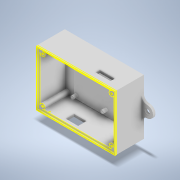
# Autodesk Inventor part: esp_housing_dsrm
Saved by Autodesk Inventor 2022.2 (Build 262287030, 287C)
## iProperties
Created: 2023-01-11
Part Number: esp_housing_dsrm
Material: Generic
Document SubType Name: Modeling
Designer: Ritchie
Density: 1 g/cm^3
Appearance: Default
Author: Ritchie
Autodesk Inventor part; units mm, degrees
ref_plane "YZ Plane" through (0, 0, 0) normal (1, 0, 0) x (0, 1, 0)
ref_plane "XZ Plane" through (0, 0, 0) normal (0, 1, 0) x (-1, 0, 0)
ref_plane "XY Plane" through (0, 0, 0) normal (0, 0, 1) x (1, 0, 0)
sketch "Sketch1" plane through (0, 0, 0) normal (0, 0, 1) x (1, 0, 0)
  line L0 (0, 0) -> (65.024, 0)
  line L1 (65.024, 0) -> (65.024, 56.742)
  line L2 (65.024, 56.742) -> (0, 56.742)
  line L3 (0, 56.742) -> (0, 0)
  point P0 (2.746, 53.796)
  point P1 (62.746, 53.796)
  point P2 (62.746, 3.796)
  point P3 (2.746, 3.796)
  point P4 (38.746, 53.796)
  point P5 (38.746, 6.796)
  dimension "d0" = 56.742
  dimension "d1" = 65.024
  dimension "d2" = 53.796
  dimension "d3" = 2.746
  dimension "d4" = 62.746
  dimension "d5" = 3.796
  dimension "d6" = 38.746
  dimension "d7" = 6.796
  dimension "d8" = 53.796
  dimension "d9" = 38.746
  constraints: 8 end point, 2 horizontal alignment, 2 parallel, 2 vertical alignment, 1 horizontal, 1 perpendicular
  measures "d0" distance of L2.end L0.start
  measures "d1" distance of L1.end L2.end
  measures "d2" distance from line of point (2.746, 53.796) L0
  measures "d3" distance from line of L3 point (2.746, 53.796)
  measures "d4" distance from line of L3 point (62.746, 53.796)
  measures "d5" distance from line of L0 point (2.746, 3.796)
  measures "d6" distance from line of point (38.746, 6.796) L3
  measures "d7" distance from line of L0 point (38.746, 6.796)
  measures "d8" distance from line of L0 point (38.746, 53.796)
  measures "d9" distance from line of L3 point (38.746, 53.796)
extrude "Extrusion1" add sketch "Sketch1" along normal blind 4
sketch "Sketch2" plane through (0, 0, 4) normal (0, 0, 1) x (1, 0, 0)
  circle A0 centre (2.746, 53.796) radius 2
  circle A1 centre (62.746, 53.796) radius 2
  circle A2 centre (38.746, 53.796) radius 2
  circle A3 centre (38.746, 6.796) radius 2
  circle A4 centre (2.746, 3.796) radius 2
  circle A5 centre (62.746, 3.796) radius 2
  point P0 (0, 0)
  dimension "d12" = 4
  dimension "d13" = 4
  dimension "d14" = 4
  dimension "d15" = 4
  dimension "d16" = 4
  dimension "d17" = 4
  constraints: 6 centre point, 6 coincident
  measures "d12" diameter of A0
  measures "d13" diameter of A1
  measures "d14" diameter of A2
  measures "d15" diameter of A3
  measures "d16" diameter of A4
  measures "d17" diameter of A5
extrude "Extrusion2" add sketch "Sketch2" along normal blind 5
sketch "Sketch3" plane through (2.746, 53.796, 9) normal (0, 0, 1) x (1, 0, 0)
  point P0 (-2.746, -53.796)
  point P1 (60, 0)
  point P2 (0, 0)
  point P3 (0, -50)
  point P4 (60, -50)
  point P5 (36, 0)
  point P6 (36, -47)
hole "Hole1" at (2.746, 53.796, 9) at (2.746, 3.796, 9) at (38.746, 53.796, 9) at (38.746, 6.796, 9) at (62.746, 53.796, 9) at (62.746, 3.796, 9) direction (0, 0, -1) diameter 1.5 depth 8
sketch "Sketch4" plane through (0, 0, 0) normal (0, 0, -1) x (-1, 0, 0)
  line L0 (-80.024, 61.742) -> (15, 61.742)
  line L1 (15, 61.742) -> (15, -5)
  line L2 (15, -5) -> (-80.024, -5)
  line L3 (-80.024, -5) -> (-80.024, 61.742)
  line L4 (-65.024, 0) -> (-65.024, 56.742) projected
  line L5 (-65.024, 0) -> (-65.024, 56.742) projected
  line L6 (0, 0) -> (-65.024, 0) projected
  line L7 (0, 56.742) -> (0, 0) projected
  line L8 (-65.024, 56.742) -> (0, 56.742) projected
  line L9 (-65.024, 56.742) -> (0, 56.742) projected
  line L10 (0, 0) -> (-65.024, 0) projected
  line L11 (0, 56.742) -> (0, 0) projected
  line L12 (15, 28.371) -> (-80.024, 28.371) construction
  arc A0 (15, 42.371) -> (22, 35.371) centre (22, 42.371) ccw
  arc A1 (22, 21.371) -> (15, 14.371) centre (22, 14.371) ccw
  arc A2 (22, 21.371) -> (22, 35.371) centre (22, 28.371) ccw
  line L13 (-32.512, 61.742) -> (-32.512, -5) construction
  arc A3 (-87.024, 35.371) -> (-80.024, 42.371) centre (-87.024, 42.371) ccw
  arc A4 (-80.024, 14.371) -> (-87.024, 21.371) centre (-87.024, 14.371) ccw
  arc A5 (-87.024, 35.371) -> (-87.024, 21.371) centre (-87.024, 28.371) ccw
  point P0 (-80.024, 14.371)
  point P1 (-80.024, 42.371)
  dimension "d35" = 15
  dimension "d36" = 5
  dimension "d37" = 5
  dimension "d38" = 15
  dimension "d73" = 14
  dimension "d81" = 7
  constraints: 12 end point, 12 point on circle, 10 symmetric about line, 6 centre point, 4 midpoint, 3 tangent, 2 parallel, 2 point on line, 1 horizontal, 1 perpendicular, 4 other
  measures "d35" distance between parallel lines of L1 L7
  measures "d36" distance between parallel lines of L0 L8
  measures "d37" distance between parallel lines of L2 L6
  measures "d38" distance between parallel lines of L3 L4
  measures "d73" diameter of A0
  measures "d81" radius of A2
extrude "Extrusion3" add sketch "Sketch4" against normal blind 3
sketch "Sketch5" plane through (0, 0, 3) normal (0, 0, 1) x (1, 0, 0)
  line L0 (-15, 61.742) -> (-15, -5) projected
  line L1 (80.024, 61.742) -> (-15, 61.742) projected
  line L2 (-15, -5) -> (80.024, -5) projected
  line L3 (80.024, -5) -> (80.024, 61.742) projected
  line L4 (-12, 58.742) -> (-12, -2)
  line L5 (-12, -2) -> (77.024, -2)
  line L6 (77.024, -2) -> (77.024, 58.742)
  line L7 (77.024, 58.742) -> (-12, 58.742)
  point P0 (0, 0)
  dimension "d29" = 3
  constraints: 8 end point, 3 other
  measures "d29" distance between parallel lines of L0 L4
extrude "Extrusion4" add sketch "Sketch5" along normal blind 30
sketch "Sketch6" plane through (0, 0, 33) normal (0, 0, 1) x (1, 0, 0)
  line L0 (-15, 61.742) -> (-15, -5) projected
  line L1 (80.024, 61.742) -> (-15, 61.742) projected
  line L2 (-15, -5) -> (80.024, -5) projected
  line L3 (80.024, -5) -> (80.024, 61.742) projected
  line L4 (-14, -4) -> (-14, 60.742)
  line L5 (-14, 60.742) -> (79.024, 60.742)
  line L6 (79.024, 60.742) -> (79.024, -4)
  line L7 (79.024, -4) -> (-14, -4)
  point P0 (0, 0)
  dimension "d32" = 1
  constraints: 8 end point, 3 other
  measures "d32" distance between parallel lines of L4 L0
extrude "Extrusion5" add sketch "Sketch6" along normal blind 1.5
sketch "Sketch7" plane through (-15, -5, 0) normal (-1, 0, 0) x (0, 0, 1)
  line L0 (9, 56.796) -> (9, 60.796) construction
  line L1 (9, 53) -> (9, 23)
  line L2 (3, 3) -> (33, 3) projected
  line L3 (9, 53) -> (19, 53)
  line L4 (9, 56.796) -> (9, 60.796) projected
  line L5 (9, 53) -> (19, 53) construction
  line L6 (9, 23) -> (19, 23)
  line L7 (0, 66.742) -> (0, 0) projected
  line L8 (9, 23) -> (19, 23) construction
  line L9 (19, 23) -> (19, 53)
  point P0 (0, 5)
  dimension "d39" = 20
  dimension "d40" = 50
  dimension "d41" = 10
  dimension "d42" = 0
  dimension "d43" = 10
  dimension "d44" = 0
  constraints: 12 end point, 2 collinear, 2 horizontal, 2 perpendicular, 1 vertical
  measures "d39" distance from line of L2 L1.end
  measures "d40" distance from line of L2 L1.start
  measures "d41" distance of L1.start L3.end
  measures "d42" distance between parallel lines of L3 L5
  measures "d43" distance of L1.end L6.end
  measures "d44" distance between parallel lines of L6 L8
extrude "Extrusion6" add sketch "Sketch7" against normal blind 0.1 separate body
sketch "Sketch8" plane through (-15, -5, 0) normal (0, -1, 0) x (1, 0, 0)
  line L0 (19.746, 9) -> (15.746, 9) construction
  line L1 (30, 19) -> (45, 19)
  line L2 (45, 19) -> (45, 29)
  line L3 (45, 29) -> (30, 29)
  line L4 (30, 29) -> (30, 19)
  point P0 (15, 0)
  point P1 (15, 0)
  dimension "d47" = 10
  dimension "d48" = 15
  dimension "d49" = 15
  dimension "d50" = 10
  constraints: 8 end point, 2 parallel, 1 horizontal, 1 perpendicular
  measures "d47" distance between parallel lines of L0 L1
  measures "d48" distance from line of point (15, 0) L4
  measures "d49" distance of L1.start L1.end
  measures "d50" distance of L1.end L2.end
extrude "Extrusion7" cut sketch "Sketch8" against normal blind 3 bodies 1
sketch "Sketch9" plane through (80.024, -5, 0) normal (1, 0, 0) x (0, 0, -1)
  line L0 (-4, 5) -> (-4, 61.742) construction
  line L1 (-9, 53) -> (-9, 23) construction
  line L2 (-19, 23) -> (-19, 53) construction
  line L3 (-9, 12) -> (-19, 12)
  line L4 (-19, 12) -> (-19, 27)
  line L5 (-19, 27) -> (-9, 27)
  line L6 (-9, 27) -> (-9, 12)
  line L7 (-19, 39.742) -> (-9, 39.742)
  line L8 (-9, 39.742) -> (-9, 54.742)
  line L9 (-9, 54.742) -> (-19, 54.742)
  line L10 (-19, 54.742) -> (-19, 39.742)
  point P0 (0, 5)
  dimension "d53" = 15
  dimension "d54" = 7
  dimension "d55" = 7
  dimension "d56" = 15
  constraints: 16 end point, 4 parallel, 3 collinear, 2 horizontal, 2 perpendicular, 1 point on line
  measures "d53" distance of L3.end L4.end
  measures "d54" distance from line of L3 L0.start
  measures "d55" distance from line of L9 L0.end
  measures "d56" distance between parallel lines of L9 L7
extrude "Extrusion8" [suppressed]
sketch "Sketch10" plane through (0, 0, 4) normal (0, 0, 1) x (1, 0, 0)
  line L0 (-12, 58.742) -> (-12, -2) construction
  line L1 (-12, -2) -> (77.024, -2) construction
  line L2 (77.024, -2) -> (77.024, 58.742) construction
  line L3 (77.024, 58.742) -> (-12, 58.742) construction
  line L4 (65.024, 56.742) -> (0, 56.742) construction
  line L5 (65.024, 0) -> (65.024, 56.742) construction
  line L6 (0, 0) -> (65.024, 0) construction
  line L7 (0, 56.742) -> (0, 0) construction
  line L8 (-12, -2) -> (-12, 58.742) construction
  line L9 (-12, 28.371) -> (77.024, 28.371) construction
  line L10 (77.024, -2) -> (77.024, 58.742) construction
  line L11 (-12, 58.742) -> (77.024, 58.742) construction
  line L12 (32.512, 58.742) -> (32.512, -2) construction
  line L13 (-12, -2) -> (77.024, -2) construction
  point P0 (20.012, 40.871)
  point P1 (45.012, 40.871)
  point P2 (45.012, 15.871)
  point P3 (20.012, 15.871)
  dimension "d59" = 25
  dimension "d60" = 25
  constraints: 4 end point, 4 midpoint, 2 horizontal alignment, 2 symmetric about line, 2 vertical alignment
  measures "d59" distance of point (45.012, 40.871) point (20.012, 40.871)
  measures "d60" distance of point (20.012, 15.871) point (20.012, 40.871)
hole "Hole2" [suppressed]
sketch "Sketch11" plane through (0, 0, 3) normal (0, 0, 1) x (1, 0, 0)
  arc A0 (-22, 35.371) -> (-22, 21.371) centre (-22, 28.371) ccw projected
  arc A1 (87.024, 21.371) -> (87.024, 35.371) centre (87.024, 28.371) ccw projected
  point P0 (0, 0)
  constraints: 2 coincident
hole "Hole3" at (-22, 28.371, 3) at (87.024, 28.371, 3) direction (0, 0, -1) diameter 6 end through all bodies 1
sketch "Sketch12" plane through (0, 0, 3) normal (0, 0, 1) x (1, 0, 0)
  arc A0 (-12, 55.742) -> (-9, 58.742) centre (-9, 55.742) ccw
  line L0 (-12, 58.742) -> (77.024, 58.742) projected
  line L1 (-12, 58.742) -> (-12, -2) projected
  line L2 (-12, 55.742) -> (-12, 58.742)
  line L3 (77.024, 58.742) -> (-12, 58.742) projected
  line L4 (32.512, 58.742) -> (32.512, 0) construction
  line L5 (0, 0) -> (65.024, 0) projected
  line L6 (-12, -2) -> (-12, 58.742) projected
  line L7 (-12, 28.371) -> (77.024, 28.371) construction
  line L8 (77.024, 58.742) -> (77.024, -2) projected
  line L9 (-12, 58.742) -> (-9, 58.742)
  arc A1 (74.024, 58.742) -> (77.024, 55.742) centre (74.024, 55.742) ccw
  line L10 (77.024, 55.742) -> (77.024, 58.742)
  line L11 (77.024, 58.742) -> (74.024, 58.742)
  arc A2 (-9, -2) -> (-12, 1) centre (-9, 1) ccw
  line L12 (-12, 1) -> (-12, -2)
  line L13 (-12, -2) -> (-9, -2)
  arc A3 (77.024, 1) -> (74.024, -2) centre (74.024, 1) ccw
  line L14 (77.024, 1) -> (77.024, -2)
  line L15 (77.024, -2) -> (74.024, -2)
  circle A4 centre (-9, 55.742) radius 1
  circle A5 centre (74.024, 55.742) radius 1
  circle A6 centre (-9, 1) radius 1
  circle A7 centre (74.024, 1) radius 1
  point P0 (77.024, 55.742)
  point P1 (77.024, 1)
  point P2 (-12, 1)
  dimension "d82" = 3
  dimension "d83" = 2
  constraints: 20 end point, 12 symmetric about line, 8 centre point, 8 point on circle, 4 midpoint, 2 collinear, 2 point on line, 2 tangent, 1 coincident, 6 other
  measures "d82" radius of A0
  measures "d83" diameter of A4
extrude "Extrusion9" add sketch "Sketch12" along normal up to surface (30 mm away) bodies 1
sketch "Sketch13" plane through (-15, 61.742, 0) normal (0, 1, 0) x (1, 0, 0)
  line L0 (0, 0) -> (95.024, 0) projected
  line L1 (95.024, 0) -> (95.024, -34.5) projected
  line L2 (45, -29) -> (45, -19) construction
  line L3 (45, -24) -> (72.5167, -24) construction
  line L4 (81.5167, -21.5) -> (63.5167, -21.5)
  line L5 (63.5167, -21.5) -> (63.5167, -26.5)
  line L6 (63.5167, -26.5) -> (81.5167, -26.5)
  line L7 (81.5167, -26.5) -> (81.5167, -21.5)
  line L8 (81.5167, -21.5) -> (63.5167, -26.5) construction
  line L9 (63.5167, -21.5) -> (81.5167, -26.5) construction
  point P0 (15, 0)
  dimension "d88" = 22.5073
  dimension "d89" = 18
  dimension "d90" = 5
  constraints: 14 end point, 3 midpoint, 2 horizontal, 2 parallel, 1 perpendicular
  measures "d88" distance from line of L1 L3.end
  measures "d89" distance of L6.end L5.end
  measures "d90" distance of L5.end L4.end
extrude "Extrusion10" cut sketch "Sketch13" against normal blind 10 bodies 1
sketch "Sketch14" plane through (0, 0, 34.5) normal (0, 0, 1) x (1, 0, 0)
  line L0 (-14, -4) -> (79.024, -4) projected
  line L1 (79.024, -4) -> (79.024, 60.742) projected
  line L2 (79.024, 60.742) -> (-14, 60.742) projected
  line L3 (-14, 60.742) -> (-14, -4) projected
  line L4 (-15, -5) -> (-15, 61.742) projected
  line L5 (-15, 61.742) -> (80.024, 61.742) projected
  line L6 (80.024, 61.742) -> (80.024, -5) projected
  line L7 (80.024, -5) -> (-15, -5) projected
  point P0 (0, 0)
sketch "Sketch15" plane through (0, 0, 33) normal (0, 0, 1) x (1, 0, 0)
  circle A0 centre (-9, 1) radius 1 projected
  circle A1 centre (74.024, 55.742) radius 1 projected
  circle A2 centre (-9, 55.742) radius 1 projected
  arc A3 (77.024, 1) -> (74.024, -2) centre (74.024, 1) ccw projected
  line L0 (77.024, 1) -> (77.024, 55.742) projected
  arc A4 (74.024, 58.742) -> (77.024, 55.742) centre (74.024, 55.742) ccw projected
  line L1 (74.024, 58.742) -> (-9, 58.742) projected
  arc A5 (-12, 55.742) -> (-9, 58.742) centre (-9, 55.742) ccw projected
  line L2 (-12, 55.742) -> (-12, 1) projected
  arc A6 (-9, -2) -> (-12, 1) centre (-9, 1) ccw projected
  line L3 (-9, -2) -> (74.024, -2) projected
  circle A7 centre (74.024, 1) radius 1 projected
  line L4 (-14, -4) -> (79.024, -4) projected
  line L5 (79.024, -4) -> (79.024, 60.742) projected
  line L6 (79.024, 60.742) -> (-14, 60.742) projected
  line L7 (-14, 60.742) -> (-14, -4) projected
  line L8 (-15, -5) -> (-15, 61.742) projected
  line L9 (-15, 61.742) -> (80.024, 61.742) projected
  line L10 (80.024, 61.742) -> (80.024, -5) projected
  line L11 (80.024, -5) -> (-15, -5) projected
  point P0 (0, 0)
equation "\"d13\" = d12"
equation "\"d14\" = d12"
equation "\"d15\" = d12"
equation "\"d16\" = d12"
equation "\"d17\" = d12"
equation "\"d73\" = 2 * d81"
body "Solid1"
body "Solid2"
